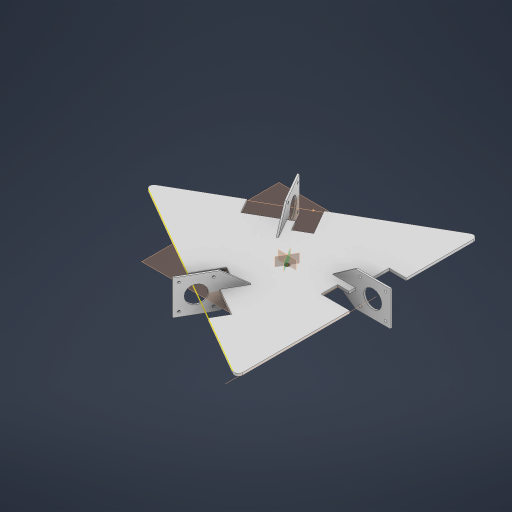
# Autodesk Inventor part: baseplate
Saved by Autodesk Inventor 2024 (Build 280153000, 153)
## iProperties
Created: 2026-03-23
Part Number: baseplate
Material: Generic
Document SubType Name: Modeling
Designer: schar
Density: 1 g/cm^3
Appearance: Default
Author: schar
Autodesk Inventor part; units mm, degrees
ref_plane "YZ Plane" through (0, 0, 0) normal (1, 0, 0) x (0, 1, 0)
ref_plane "XZ Plane" through (0, 0, 0) normal (0, 1, 0) x (-1, 0, 0)
ref_plane "XY Plane" through (0, 0, 0) normal (0, 0, 1) x (1, 0, 0)
sketch "Sketch1" plane through (0, 0, 0) normal (0, 1, 0) x (-1, 0, 0)
  line L0 (-79.1025, 145.6699) -> (165.7051, 4.3301)
  line L1 (165.7051, -4.3301) -> (-79.1025, -145.6699)
  line L2 (-86.6025, -141.3397) -> (-86.6025, 141.3397)
  arc A0 (165.7051, -4.3301) -> (165.7051, 4.3301) centre (163.2051, 0) ccw
  arc A1 (-86.6025, -141.3397) -> (-79.1025, -145.6699) centre (-81.6025, -141.3397) ccw
  arc A2 (-79.1025, 145.6699) -> (-86.6025, 141.3397) centre (-81.6025, 141.3397) ccw
  line L3 (43.3013, -75) -> (-37.0012, 64.088)
  line L4 (-86.6025, 0) -> (172.7545, 0)
  line L5 (43.3013, 75) -> (-33.1798, -57.4692)
  circle A3 centre (0, 0) radius 2.5
  point P0 (0, 0)
  point P1 (-86.6025, 150)
  point P2 (-86.6025, -150)
  dimension "d5" = 300
  dimension "d9" = 60
  dimension "d10" = 60
  dimension "d14" = 5
  dimension "d25" = 5
  constraints: 12 end point, 6 point on circle, 6 point on line, 6 tangent, 4 centre point, 3 midpoint, 3 perpendicular, 2 equal radius, 1 coincident
  measures "d5" distance of point (-86.603, -150) point (-86.603, 150)
  measures "d9" angle of L1 L0
  measures "d10" angle of L1 L2
  measures "d14" radius of A0
  measures "d25" diameter of A3
extrude "Extrusion1" add sketch "Sketch1" along normal blind 3
sketch "Sketch2" plane through (0, 3, 0) normal (0, 1, 0) x (1, 0, 0)
  point P0 (0, 0)
ref_plane "Work Plane1" through (0, 1.5, 0) normal (0, 1, 0) x (1, 0, 0)
ref_plane "Work Plane2" through (0, 3, 0) normal (0.8660254, 0, 0.5) x (0, 1, 0)
ref_plane "Work Plane3" through (0, 3, 0) normal (-0.8660254, 0, 0.5) x (0, -1, 0)
ref_plane "Work Plane4" through (0, 3, 0) normal (0, 0, 1) x (1, 0, 0)
sketch "Sketch3" plane through (0, 3, 0) normal (0, 1, 0) x (1, 0, 0)
  line L0 (86.6025, 0) -> (86.6025, 10)
  line L1 (86.6025, 10) -> (51.6025, 10)
  line L2 (121.6025, -10) -> (51.6025, -10)
  line L3 (51.6025, -10) -> (51.6025, 10)
  line L4 (51.6025, 10) -> (121.6025, 10)
  line L5 (121.6025, 10) -> (121.6025, -10)
  line L6 (121.6025, -10) -> (51.6025, 10) construction
  line L7 (51.6025, -10) -> (121.6025, 10) construction
  line L8 (92.1025, -0.5) -> (81.1025, -0.5)
  line L9 (81.1025, -0.5) -> (81.1025, 20.5)
  line L10 (81.1025, 20.5) -> (92.1025, 20.5)
  line L11 (92.1025, 20.5) -> (92.1025, -0.5)
  line L12 (92.1025, -0.5) -> (81.1025, 20.5) construction
  line L13 (81.1025, -0.5) -> (92.1025, 20.5) construction
  line L14 (86.6025, 20.5) -> (86.6025, 20.5)
  line L15 (86.6025, 20.5) -> (82.6025, 20.5)
  line L16 (82.6025, 20.5) -> (82.6025, 20.5)
  line L17 (82.6025, 20.5) -> (86.6025, 20.5)
  line L18 (86.6025, 20.5) -> (86.6025, 20.5)
  line L19 (86.6025, 10) -> (86.6025, 19)
  line L20 (86.6025, 19) -> (65.6025, 19)
  line L21 (65.6025, 19) -> (65.6025, 59)
  line L22 (65.6025, 59) -> (86.6025, 59)
  line L23 (86.6025, 59) -> (86.6025, 19)
  line L24 (65.6025, 19) -> (65.6025, 10)
  point P0 (0, 0)
  point P1 (81.1025, 10)
  point P2 (81.1025, 19)
  point P3 (92.1025, 10)
  dimension "d17" = 10
  dimension "d18" = 35
  dimension "d19" = 11
  dimension "d20" = 21
  dimension "d23" = 0
  dimension "d27" = 4
  dimension "d28" = 9
  dimension "d29" = 21
  dimension "d30" = 40
  dimension "d31" = 0
  dimension "d32" = 121.6025
  dimension "d33" = 10
  dimension "d34" = 29.5
  dimension "d35" = 11.1262
  dimension "d36" = 35
  dimension "d37" = 0
  dimension "d38" = 39
  dimension "d39" = 10.5
  dimension "d40" = 40.5
  dimension "d41" = 16.758
  dimension "d42" = 40.5
  dimension "d43" = 0
  constraints: 50 end point, 11 perpendicular, 7 parallel, 5 midpoint, 2 horizontal, 2 point on line, 1 collinear
  measures "d17" distance of L0.start L0.end
  measures "d18" distance of L0.end L1.end
  measures "d19" distance of L8.start L8.end
  measures "d20" distance of L8.end L9.end
  measures "d23" distance of L14.start L14.end
  measures "d27" distance of L16.end L17.end
  measures "d28" distance of L0.end L19.end
  measures "d29" distance of L19.end L20.end
  measures "d30" distance of L20.end L21.end
  measures "d31" distance between parallel lines of L10 L17
  measures "d32" distance from line of point (0, 0) L5
  measures "d33" distance from line of point (0, 0) L2
  measures "d34" distance from line of point (92.103, 10) L5
  measures "d35" distance from line of point (92.103, 10) L6
  measures "d36" distance from line of point (86.603, 20.5) L5
  measures "d37" distance from line of point (86.603, 20.5) L10
  measures "d38" distance from line of point (82.603, 20.5) L5
  measures "d39" distance from line of point (82.603, 20.5) L4
  measures "d40" distance from line of point (81.103, 19) L5
  measures "d41" distance from line of point (81.103, 19) L6
  measures "d42" distance from line of point (81.103, 10) L5
  measures "d43" distance from line of point (81.103, 10) L4
extrude "Extrusion2" cut sketch "Sketch3" against normal blind 3
sketch "Sketch4" plane through (0, 3, 0) normal (0, 1, 0) x (1, 0, 0)
  point P0 (0, 0)
ref_plane "Work Plane5" through (0, 1.5, 0) normal (0, 1, 0) x (1, 0, 0)
ref_plane "Work Plane6" through (51.6025, 3, -19) normal (0, 0, 1) x (1, 0, 0)
sketch "Sketch6" plane through (0, 3, 0) normal (0, 1, 0) x (1, 0, 0)
  point P0 (0, 0)
sketch "Sketch7" plane through (0, 1.5, 0) normal (0, 1, 0) x (1, 0, 0)
  line L0 (-43.3013, 75) -> (-51.9615, 70)
  line L1 (-51.9615, 70) -> (-34.4615, 39.6891)
  line L2 (-52.141, 110.3109) -> (-17.141, 49.6891)
  line L3 (-17.141, 49.6891) -> (-34.4615, 39.6891)
  line L4 (-34.4615, 39.6891) -> (-69.4615, 100.3109)
  line L5 (-69.4615, 100.3109) -> (-52.141, 110.3109)
  line L6 (-52.141, 110.3109) -> (-34.4615, 39.6891) construction
  line L7 (-17.141, 49.6891) -> (-69.4615, 100.3109) construction
  line L8 (-45.6183, 80.0131) -> (-40.1183, 70.4869)
  line L9 (-40.1183, 70.4869) -> (-58.3048, 59.9869)
  line L10 (-58.3048, 59.9869) -> (-63.8048, 69.5131)
  line L11 (-63.8048, 69.5131) -> (-45.6183, 80.0131)
  line L12 (-45.6183, 80.0131) -> (-58.3048, 59.9869) construction
  line L13 (-40.1183, 70.4869) -> (-63.8048, 69.5131) construction
  line L14 (-61.0548, 64.75) -> (-61.0548, 64.75)
  line L15 (-61.0548, 64.75) -> (-59.0548, 61.2859)
  line L16 (-59.0548, 61.2859) -> (-59.0548, 61.2859)
  line L17 (-59.0548, 61.2859) -> (-61.0548, 64.75)
  line L18 (-61.0548, 64.75) -> (-61.0548, 64.75)
  line L19 (-51.9615, 70) -> (-59.7558, 65.5)
  line L20 (-59.7558, 65.5) -> (-49.2558, 47.3135)
  line L21 (-49.2558, 47.3135) -> (-83.8968, 27.3135)
  line L22 (-83.8968, 27.3135) -> (-94.3968, 45.5)
  line L23 (-94.3968, 45.5) -> (-59.7558, 65.5)
  line L24 (-49.2558, 47.3135) -> (-41.4615, 51.8135)
  line L25 (-25.5477, -85.25) -> (-25.5477, -85.25)
  line L26 (-25.5477, -85.25) -> (-25.5477, -85.25)
  line L27 (-34.641, -80) -> (-26.8468, -84.5)
  line L28 (-23.5477, -81.7859) -> (-25.5477, -85.25)
  line L29 (-22.7977, -80.4869) -> (-28.2977, -90.0131)
  line L30 (-28.2977, -90.0131) -> (-46.4843, -79.5131)
  line L31 (-40.9843, -69.9869) -> (-28.2977, -90.0131) construction
  line L32 (-46.4843, -79.5131) -> (-40.9843, -69.9869)
  line L33 (-46.4843, -79.5131) -> (-22.7977, -80.4869) construction
  line L34 (-40.9843, -69.9869) -> (-22.7977, -80.4869)
  line L35 (-17.141, -49.6891) -> (-52.141, -110.3109)
  line L36 (-69.4615, -100.3109) -> (-17.141, -49.6891) construction
  line L37 (-69.4615, -100.3109) -> (-34.4615, -39.6891)
  line L38 (-34.4615, -39.6891) -> (-52.141, -110.3109) construction
  line L39 (-16.3468, -66.3135) -> (-24.141, -61.8135)
  line L40 (-34.641, -80) -> (-17.141, -49.6891)
  line L41 (-34.4615, -39.6891) -> (-17.141, -49.6891)
  line L42 (-25.5477, -85.25) -> (-23.5477, -81.7859)
  line L43 (-26.8468, -84.5) -> (-16.3468, -66.3135)
  line L44 (7.7942, -104.5) -> (-26.8468, -84.5)
  line L45 (-16.3468, -66.3135) -> (18.2942, -86.3135)
  line L46 (18.2942, -86.3135) -> (7.7942, -104.5)
  line L47 (-23.5477, -81.7859) -> (-23.5477, -81.7859)
  line L48 (-52.141, -110.3109) -> (-69.4615, -100.3109)
  line L49 (-43.3013, -75) -> (-34.641, -80)
  point P0 (0, 0)
  point P1 (-43.3013, 75)
  point P2 (-43.3013, -75)
  point P3 (-37.391, -84.7631)
  dimension "d45" = 10
  dimension "d46" = 35
  dimension "d47" = 11
  dimension "d48" = 21
  dimension "d50" = 4
  dimension "d51" = 9
  dimension "d52" = 21
  dimension "d53" = 40
  dimension "d59" = 10
  dimension "d60" = 35
  dimension "d61" = 11
  dimension "d62" = 21
  dimension "d63" = 4
  dimension "d64" = 9
  dimension "d65" = 21
  dimension "d66" = 40
  constraints: 100 end point, 22 perpendicular, 14 parallel, 10 midpoint, 4 point on line, 2 collinear
  measures "d45" distance of L0.start L19.start
  measures "d46" distance of L19.start L4.start
  measures "d47" distance of L11.end L13.start
  measures "d48" distance of L13.start L10.start
  measures "d50" distance of L17.start L18.start
  measures "d51" distance of L19.start L19.end
  measures "d52" distance of L19.end L24.start
  measures "d53" distance of L24.start L21.end
  measures "d59" distance of L49.start L27.start
  measures "d60" distance of L27.start L35.start
  measures "d61" distance of L33.start L31.start
  measures "d62" distance of L31.start L29.start
  measures "d63" distance of L47.end L26.start
  measures "d64" distance of L27.start L27.end
  measures "d65" distance of L27.end L43.end
  measures "d66" distance of L43.end L46.start
extrude "Extrusion3" cut sketch "Sketch7" along normal mid plane 3 contours L1 L9 L8 L11 L4 L5 L2 L3 | L24 L20 L9 L1 | L9 L20 L19 L1 | L1 L4 L11 L8 L9 | L21 L22 L23 L10 L9 L20 | L9 L10 L23 L20 | L35 L34 L43 L27 | L35 L30 L32 L34 | L27 L44 L29 L30 L35 | L43 L34 L29 L28 L44 | L35 L39 L43 L34 | L34 L32 L30 L35 L48 L37 L41 | L43 L45 L46 L44 L28 L29 L34
sketch "Sketch9" plane through (0, 3, 0) normal (0, 1, 0) x (1, 0, 0)
  line L0 (-165.7051, -4.3301) -> (79.1025, -145.6699) projected
  point P0 (0, 0)
  point P1 (-43.3013, -75)
  constraints: 1 midpoint
ref_plane "Work Plane7" through (-42.2558, 0, -35.1891) normal (0.8660254, 0, -0.5) x (-0.5, 0, -0.8660254)
ref_plane "Work Plane8" through (-9.3468, 0, 54.1891) normal (-0.8660254, 0, -0.5) x (-0.5, 0, 0.8660254)
sketch "Sketch10" plane through (-9.3468, 0, 54.1891) normal (-0.8660254, 0, -0.5) x (-0.5, 0, 0.8660254)
  line L0 (14, 0) -> (14, 3) projected
  line L1 (14, 1.5) -> (14, 17)
  line L2 (14, 17) -> (19.65, 17)
  circle A0 centre (19.65, 17) radius 1.5
  line L3 (19.65, 17) -> (50.65, 17)
  line L4 (50.65, 17) -> (50.65, -14)
  line L5 (50.65, -14) -> (19.65, -14)
  line L6 (19.65, -14) -> (19.65, 17)
  line L7 (14, 1.5) -> (14, 22.65)
  line L8 (19.65, 17) -> (19.65, 22.65)
  circle A1 centre (19.65, -14) radius 1.5
  circle A2 centre (50.65, -14) radius 1.5
  circle A3 centre (50.65, 17) radius 1.5
  line L9 (50.65, -14) -> (56.3, -14)
  line L10 (56.3, -14) -> (56.3, -19.65)
  line L11 (14, 22.65) -> (56.3, 22.65)
  line L12 (56.3, 22.65) -> (56.3, -19.65)
  line L13 (56.3, -19.65) -> (14, -19.65)
  line L14 (14, -19.65) -> (14, 22.65)
  line L15 (14, 1.5) -> (-16, 1.5)
  line L16 (-16, 1.5) -> (14, 22.65)
  line L17 (-16, 1.5) -> (14, -19.65)
  line L18 (35.15, 17) -> (35.15, -14)
  line L19 (19.65, 1.5) -> (50.65, 1.5)
  circle A4 centre (35.15, 1.5) radius 11
  point P0 (-51.6025, 0)
  point P1 (56.3, -14)
  dimension "d70" = 15.5
  dimension "d71" = 5.65
  dimension "d72" = 3
  dimension "d73" = 31
  dimension "d74" = 31
  dimension "d75" = 21.15
  dimension "d76" = 5.65
  dimension "d77" = 90
  dimension "d78" = 90
  dimension "d79" = 3
  dimension "d80" = 3
  dimension "d81" = 3
  dimension "d82" = 5.65
  dimension "d83" = 5.65
  dimension "d84" = 30
  dimension "d85" = 22
  constraints: 38 end point, 6 midpoint, 5 centre point, 4 coincident, 4 horizontal, 4 parallel, 4 perpendicular, 2 vertical
  measures "d70" distance of L1.start L1.end
  measures "d71" distance of L1.end L2.end
  measures "d72" diameter of A0
  measures "d73" distance of L4.end L5.end
  measures "d74" distance of L3.end L4.end
  measures "d75" distance of L1.start L7.end
  measures "d76" distance of L3.start L8.end
  measures "d77" angle of L2 L0
  measures "d78" angle of L1 L3
  measures "d79" diameter of A1
  measures "d80" diameter of A2
  measures "d81" diameter of A3
  measures "d82" distance of L9.start L9.end
  measures "d83" distance of L9.end L10.end
  measures "d84" distance of L1.start L15.end
  measures "d85" diameter of A4
extrude "Extrusion4" add sketch "Sketch10" along normal mid plane 2 contours L14 L17 L15 L0 | L0 L1 L2 A0 L6 A1 L5 A2 L9 L10 L13 L14 | L15 L16 L7 L1 L0 | L7 L11 L8 A0 L2 | L9 A2 L4 A3 L3 A0 L8 L11 L12 | A0 L3 L18 A4 L19 L6 | A2 L5 L18 A4 L19 L4 | L19 A4 L18 L5 A1 L6 | L19 A4 L18 L3 A3 L4
sketch "Sketch11" plane through (-42.2558, 0, -35.1891) normal (0.8660254, 0, -0.5) x (-0.5, 0, -0.8660254)
  line L0 (14, 0) -> (14, 3) projected
  line L1 (14, 0) -> (14, 3)
  line L2 (14, 1.5) -> (14, 17)
  line L3 (14, 17) -> (19.65, 17)
  circle A0 centre (19.65, 17) radius 1.5
  line L4 (19.65, 17) -> (50.65, 17)
  line L5 (50.65, 17) -> (50.65, -14)
  line L6 (50.65, -14) -> (19.65, -14)
  line L7 (19.65, -14) -> (19.65, 17)
  line L8 (14, 1.5) -> (14, 22.65)
  line L9 (19.65, 17) -> (19.65, 22.65)
  circle A1 centre (19.65, -14) radius 1.5
  circle A2 centre (50.65, -14) radius 1.5
  circle A3 centre (50.65, 17) radius 1.5
  line L10 (50.65, -14) -> (56.3, -14)
  line L11 (56.3, -14) -> (56.3, -19.65)
  line L12 (14, 22.65) -> (56.3, 22.65)
  line L13 (56.3, 22.65) -> (56.3, -19.65)
  line L14 (56.3, -19.65) -> (14, -19.65)
  line L15 (14, -19.65) -> (14, 22.65)
  line L16 (14, 1.5) -> (-16, 1.5)
  line L17 (-16, 1.5) -> (14, 22.65)
  line L18 (-16, 1.5) -> (14, -19.65)
  line L19 (35.15, 17) -> (35.15, -14)
  line L20 (19.65, 1.5) -> (50.65, 1.5)
  circle A4 centre (35.15, 1.5) radius 11
  point P0 (-51.6025, 0)
  point P1 (14, 1.5)
  dimension "d88" = 15.5
  dimension "d89" = 5.65
  dimension "d90" = 3
  dimension "d91" = 31
  dimension "d92" = 31
  dimension "d93" = 21.15
  dimension "d94" = 5.65
  dimension "d95" = 90
  dimension "d96" = 90
  dimension "d97" = 3
  dimension "d98" = 3
  dimension "d99" = 3
  dimension "d100" = 5.65
  dimension "d101" = 5.65
  dimension "d102" = 30
  dimension "d103" = 22
  constraints: 40 end point, 7 midpoint, 5 centre point, 4 coincident, 4 horizontal, 4 parallel, 4 perpendicular, 2 vertical
  measures "d88" distance of L16.start L2.end
  measures "d89" distance of L2.end L3.end
  measures "d90" diameter of A0
  measures "d91" distance of L5.end L7.start
  measures "d92" distance of L4.end L5.end
  measures "d93" distance of L16.start L17.end
  measures "d94" distance of L7.end L9.end
  measures "d95" angle of L3 L1
  measures "d96" angle of L2 L4
  measures "d97" diameter of A1
  measures "d98" diameter of A2
  measures "d99" diameter of A3
  measures "d100" distance of L10.start L10.end
  measures "d101" distance of L10.end L14.start
  measures "d102" distance of L16.start L17.start
  measures "d103" diameter of A4
extrude "Extrusion5" add sketch "Sketch11" along normal mid plane 2 contours L15 L18 L16 L0 | L0 L2 L3 A0 L7 A1 L6 A2 L10 L11 L14 L15 | L16 L17 L8 L2 L0 | L8 L12 L9 A0 L3 | L10 A2 L5 A3 L4 A0 L9 L12 L13 | A0 L4 L19 A4 L20 L7 | A2 L6 L19 A4 L20 L5 | L20 A4 L19 L6 A1 L7 | L20 A4 L19 L4 A3 L5
sketch "Sketch12" plane through (51.6025, 3, -19) normal (0, 0, 1) x (1, 0, 0)
  line L0 (14, -3) -> (14, 0)
  line L1 (-16, -1.5) -> (14, 19.65)
  line L2 (14, -1.5) -> (-16, -1.5)
  line L3 (-16, -1.5) -> (14, -22.65)
  line L4 (14, -3) -> (14, 0)
  line L5 (14, -1.5) -> (14, 14)
  circle A0 centre (19.65, -17) radius 1.5
  line L6 (14, -22.65) -> (14, 19.65)
  line L7 (14, -1.5) -> (14, 19.65)
  line L8 (14, 14) -> (19.65, 14)
  line L9 (19.65, -17) -> (19.65, 14)
  line L10 (19.65, 14) -> (19.65, 19.65)
  circle A1 centre (19.65, 14) radius 1.5
  line L11 (35.15, 14) -> (35.15, -17)
  line L12 (19.65, 14) -> (50.65, 14)
  line L13 (50.65, 14) -> (50.65, -17)
  line L14 (50.65, -17) -> (19.65, -17)
  circle A2 centre (35.15, -1.5) radius 11
  line L15 (19.65, -1.5) -> (50.65, -1.5)
  line L16 (14, 19.65) -> (56.3, 19.65)
  line L17 (56.3, -22.65) -> (14, -22.65)
  circle A3 centre (50.65, 14) radius 1.5
  line L18 (56.3, 19.65) -> (56.3, -22.65)
  circle A4 centre (50.65, -17) radius 1.5
  line L19 (50.65, -17) -> (56.3, -17)
  line L20 (56.3, -17) -> (56.3, -22.65)
  line L21 (14, 0) -> (14, -3) projected
  point P0 (-51.6025, -3)
  point P1 (14, -1.5)
  point P2 (14, -1.5)
  point P3 (56.3, -17)
  dimension "d106" = 15.5
  dimension "d107" = 5.65
  dimension "d108" = 3
  dimension "d109" = 31
  dimension "d110" = 31
  dimension "d111" = 21.15
  dimension "d112" = 5.65
  dimension "d113" = 90
  dimension "d114" = 90
  dimension "d115" = 3
  dimension "d116" = 3
  dimension "d117" = 3
  dimension "d118" = 5.65
  dimension "d119" = 5.65
  dimension "d120" = 30
  dimension "d121" = 22
  constraints: 42 end point, 8 midpoint, 5 centre point, 4 coincident, 4 horizontal, 4 parallel, 4 perpendicular, 2 vertical
  measures "d106" distance of L2.start L8.start
  measures "d107" distance of L8.start L8.end
  measures "d108" diameter of A1
  measures "d109" distance of L14.start L14.end
  measures "d110" distance of L13.start L14.start
  measures "d111" distance of L2.start L1.end
  measures "d112" distance of L10.start L10.end
  measures "d113" angle of L8 L4
  measures "d114" angle of L5 L12
  measures "d115" diameter of A0
  measures "d116" diameter of A4
  measures "d117" diameter of A3
  measures "d118" distance of L19.start L20.start
  measures "d119" distance of L20.start L20.end
  measures "d120" distance of L2.start L1.start
  measures "d121" diameter of A2
extrude "Extrusion6" add sketch "Sketch12" along normal mid plane 2 contours L6 L3 L2 L0 | L0 L5 L8 A1 L9 A0 L14 A4 L19 L18 L17 L6 | L2 L1 L6 L5 L0 | L6 L16 L10 A1 L8 | L19 A4 L13 A3 L12 A1 L10 L16 L18 | A1 L12 L11 A2 L15 L9 | A4 L14 L11 A2 L15 L13 | L15 A2 L11 L14 A0 L9 | L15 A2 L11 L12 A3 L13
sketch "Sketch13" plane through (0, 3, 0) normal (0, 1, 0) x (1, 0, 0)
  circle A0 centre (0, 0) radius 2.5
  dimension "d124" = 5
  constraints: 1 centre point, 1 coincident
  measures "d124" diameter of A0
extrude "Extrusion7" cut sketch "Sketch13" against normal through all
body "Solid1"
